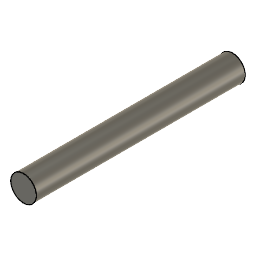
Eje 7mm (Autodesk Fusion 360 design; units mm, degrees)
Autodesk Fusion 360 part; units mm, degrees
sketch "Boceto1" plane through (0, 0, 0) normal (0, 1, 0) x (1, 0, 0)
  circle A0 centre (0, 0) radius 3.5
  dimension "d1" = 7
  constraint coincident A0.centre origin
  measures "d1" diameter of A0
extrude "Extruir1" add sketch "Boceto1" along normal blind 65
ref_plane "PlanoDeObra1" through (0, 2.15, 0) normal (0, -1, 0) x (-1, 0, 0)
sketch "Boceto2" plane through (0, 2.15, 0) normal (0, -1, 0) x (-1, 0, 0)
  circle A0 centre (0, 0) radius 3
  circle A1 centre (0, 0) radius 3.5
  dimension "d5" = 6
  dimension "d6" = 7
  constraint coincident A0.centre A1.centre
  measures "d5" diameter of A0
  measures "d6" diameter of A1
extrude "Extruir2" cut sketch "Boceto2" against normal blind 0.85
ref_plane "PlanoDeObra2" through (0, 62.85, 0) normal (0, 1, 0) x (1, 0, 0)
sketch "Boceto3" plane through (0, 62.85, 0) normal (0, 1, 0) x (1, 0, 0)
  circle A0 centre (0, 0) radius 3
  circle A1 centre (0, 0) radius 3.5
  dimension "d10" = 6
  dimension "d11" = 7
  constraint coincident A0.centre A1.centre
  measures "d10" diameter of A0
  measures "d11" diameter of A1
extrude "Extruir3" cut sketch "Boceto3" against normal blind 0.85
move_face "CarasDesfase1" offset -4 2 faces at (0.555, 0, 0.9381) (0.555, 65, 0.9381)
